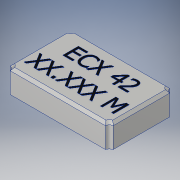
# Autodesk Inventor part: Crystal_ECX-42
Saved by Autodesk Inventor 2017 (Build 210142000, 142)
## iProperties
Created: 2016-08-15
Part Number: Crystal_ECX-42
Material: Aluminum 6061
Document SubType Name: Modeling
Designer: Bradley
Density: 2.7 g/cm^3
Appearance: Aluminum - Flat
Author: Bradley
Autodesk Inventor part; units mm, degrees
ref_plane "YZ Plane" through (0, 0, 0) normal (1, 0, 0) x (0, 1, 0)
ref_plane "XZ Plane" through (0, 0, 0) normal (0, 1, 0) x (-1, 0, 0)
ref_plane "XY Plane" through (0, 0, 0) normal (0, 0, 1) x (1, 0, 0)
sketch "Sketch1" plane through (0, 0, 0) normal (0, 1, 0) x (-1, 0, 0)
  line L0 (-2, 1.25) -> (2, 1.25)
  line L1 (2, 1.25) -> (2, -1.25)
  line L2 (2, -1.25) -> (-2, -1.25)
  line L3 (-2, -1.25) -> (-2, 1.25)
  line L4 (-2, 1.25) -> (2, -1.25) construction
  line L5 (2, 1.25) -> (-2, -1.25) construction
  arc A0 (2, -1.1) -> (1.85, -1.25) centre (2, -1.25) ccw
  arc A1 (-1.85, -1.25) -> (-2, -1.1) centre (-2, -1.25) ccw
  arc A2 (-2, 1.1) -> (-1.85, 1.25) centre (-2, 1.25) ccw
  arc A3 (1.85, 1.25) -> (2, 1.1) centre (2, 1.25) ccw
  point P0 (0, 0)
  dimension "d0" = 4
  dimension "d1" = 2.5
  dimension "d4" = 0.15
  constraints: 12 end point, 8 point on circle, 8 point on line, 4 centre point, 4 coincident, 3 equal radius, 2 midpoint, 2 parallel, 1 horizontal, 1 perpendicular
  measures "d0" distance of L1.end L2.end
  measures "d1" distance of L0.end L1.end
  measures "d4" radius of A0
extrude "Extrusion1" add sketch "Sketch1" along normal mid plane 0.9 contours L0 A3 L1 A0 L2 A1 L3 A2
chamfer "Chamfer1" distance 0.1 angle 45 8 edges at (0, 0.45, 1.25) (-1.8939, 0.45, 1.1439) (-2, 0.45, 0) (-1.8939, 0.45, -1.1439) (0, 0.45, -1.25) (1.8939, 0.45, -1.1439) (2, 0.45, 0) (1.8939, 0.45, 1.1439)
sketch "Sketch2" plane through (0, -0.45, 0) normal (0, -1, 0) x (1, 0, 0)
  line L0 (-2, 1.1) -> (-2, -1.1) projected
  arc A0 (-1.85, -1.25) -> (-2, -1.1) centre (-2, -1.25) ccw projected
  line L1 (-1.85, -1.25) -> (1.85, -1.25) projected
  arc A1 (2, -1.1) -> (1.85, -1.25) centre (2, -1.25) ccw projected
  line L2 (2, -1.1) -> (2, 1.1) projected
  arc A2 (1.85, 1.25) -> (2, 1.1) centre (2, 1.25) ccw projected
  line L3 (1.85, 1.25) -> (-1.85, 1.25) projected
  arc A3 (-2, 1.1) -> (-1.85, 1.25) centre (-2, 1.25) ccw projected
  arc A4 (-1.85, -1.25) -> (-2, -1.1) centre (-2, -1.25) ccw projected
  line L4 (-1.9612, -1.1051) -> (-1.9, -1.0439)
  line L5 (-1.9, 1.0439) -> (-1.9612, 1.1051)
  arc A5 (-2, 1.1) -> (-1.85, 1.25) centre (-2, 1.25) ccw projected
  line L6 (-1.8551, 1.2112) -> (-1.7939, 1.15)
  line L7 (-1.7939, 1.15) -> (-1, 1.15)
  line L8 (-1, -1.15) -> (-1.7939, -1.15)
  line L9 (-1.7939, -1.15) -> (-1.8551, -1.2112)
  arc A6 (1.85, 1.25) -> (2, 1.1) centre (2, 1.25) ccw projected
  line L10 (1.8551, 1.2112) -> (1.7939, 1.15)
  line L11 (1.7939, 1.15) -> (1, 1.15)
  line L12 (1, -1.15) -> (1.7939, -1.15)
  line L13 (1.7939, -1.15) -> (1.8551, -1.2112)
  arc A7 (2, -1.1) -> (1.85, -1.25) centre (2, -1.25) ccw projected
  line L14 (1.9612, -1.1051) -> (1.9, -1.0439)
  line L15 (1.9, 1.0439) -> (1.9612, 1.1051)
  line L16 (-2, 1.25) -> (-1.8939, 1.1439) construction
  line L17 (1.85, 1.25) -> (-1.85, 1.25) construction
  line L18 (-2, -1.25) -> (-1.8939, -1.1439) construction
  line L19 (-1.9, 1.0439) -> (-1.9, 0.35)
  line L20 (-1.9, 0.35) -> (-1, 0.35)
  line L21 (-1, 0.35) -> (-1, 1.15)
  line L22 (-1.9, -1.0439) -> (-1.9, -0.35)
  line L23 (-1.9, -0.35) -> (-1, -0.35)
  line L24 (-1, -0.35) -> (-1, -1.15)
  line L25 (1.9, -1.0439) -> (1.9, -0.35)
  line L26 (1.9, -0.35) -> (1, -0.35)
  line L27 (1, -0.35) -> (1, -1.15)
  line L28 (1.9, 1.0439) -> (1.9, 0.35)
  line L29 (1.9, 0.35) -> (1, 0.35)
  line L30 (1, 1.15) -> (1, 0.35)
  point P0 (0, 0)
  dimension "d9" = 0.15
  dimension "d15" = 2
  dimension "d16" = 0.7
  dimension "d17" = 0.8
  constraints: 52 end point, 15 equal length, 15 point on circle, 9 point on line, 8 parallel, 8 perpendicular, 1 collinear, 1 vertical, 1 other
  measures "d9" distance between parallel lines of L5 L6
  measures "d15" distance between parallel lines of L30 L21
  measures "d16" distance between parallel lines of L26 L29
  measures "d17" distance of L11.end L29.end
sketch "Sketch3" plane through (0, 0.45, 0) normal (0, 1, 0) x (1, 0, 0)
  line L0 (-1.7709, 1.15) -> (1.7709, 1.15) projected
  arc A0 (-1.9, 1.0209) -> (-1.7709, 1.15) centre (-2, 1.25) ccw projected
  line L1 (-1.9, -1.0209) -> (-1.9, 1.0209) projected
  arc A1 (-1.7709, -1.15) -> (-1.9, -1.0209) centre (-2, -1.25) ccw projected
  line L2 (1.7709, -1.15) -> (-1.7709, -1.15) projected
  arc A2 (1.9, -1.0209) -> (1.7709, -1.15) centre (2, -1.25) ccw projected
  line L3 (1.9, 1.0209) -> (1.9, -1.0209) projected
  arc A3 (1.7709, 1.15) -> (1.9, 1.0209) centre (2, 1.25) ccw projected
  line L4 (1.9, 1.0209) -> (1.9, -1.0209) construction
  line L5 (1.9, 0.1868) -> (-1.9, 0.1868) construction
  line L6 (-1.237, 0.1868) -> (-1.237, 0.7868)
  line L7 (-1.237, 0.7868) -> (-0.8616, 0.7868)
  line L8 (-0.8616, 0.7868) -> (-0.8616, 0.7158)
  line L9 (-0.8616, 0.7158) -> (-1.1572, 0.7158)
  line L10 (-1.1572, 0.7158) -> (-1.1572, 0.5514)
  line L11 (-1.1572, 0.5514) -> (-0.8815, 0.5514)
  line L12 (-0.8815, 0.5514) -> (-0.8815, 0.4804)
  line L13 (-0.8815, 0.4804) -> (-1.1572, 0.4804)
  line L14 (-1.1572, 0.4804) -> (-1.1572, 0.2577)
  line L15 (-1.1572, 0.2577) -> (-0.8616, 0.2577)
  line L16 (-0.8616, 0.2577) -> (-0.8616, 0.1868)
  line L17 (-0.8616, 0.1868) -> (-1.237, 0.1868)
  spline S0 degree 2 poles (-0.5397, 0.1761) (-0.5981, 0.1761) (-0.6968, 0.2154) (-0.7327, 0.2548) knots 0 0 0 1 2 2 2
  spline S1 degree 2 poles (-0.7327, 0.2548) (-0.7687, 0.2937) (-0.8081, 0.4104) (-0.8081, 0.4863) knots 0 0 0 1 2 2 2
  spline S2 degree 2 poles (-0.8081, 0.4863) (-0.8081, 0.5616) (-0.7697, 0.6735) (-0.7332, 0.7148) knots 0 0 0 1 2 2 2
  spline S3 degree 2 poles (-0.7332, 0.7148) (-0.6972, 0.7552) (-0.599, 0.7975) (-0.5382, 0.7975) knots 0 0 0 1 2 2 2
  spline S4 degree 2 poles (-0.5382, 0.7975) (-0.5081, 0.7975) (-0.4551, 0.7887) (-0.4327, 0.7819) knots 0 0 0 1 2 2 2
  spline S5 degree 2 poles (-0.4327, 0.7819) (-0.4133, 0.7756) (-0.3729, 0.7576) (-0.353, 0.7469) knots 0 0 0 1 2 2 2
  line L18 (-0.353, 0.7469) -> (-0.353, 0.6506)
  line L19 (-0.353, 0.6506) -> (-0.3593, 0.6506)
  spline S6 degree 2 poles (-0.3593, 0.6506) (-0.37, 0.6603) (-0.4031, 0.6876) (-0.4269, 0.7007) knots 0 0 0 1 2 2 2
  spline S7 degree 2 poles (-0.4269, 0.7007) (-0.4498, 0.7133) (-0.5037, 0.7294) (-0.5387, 0.7294) knots 0 0 0 1 2 2 2
  spline S8 degree 2 poles (-0.5387, 0.7294) (-0.5771, 0.7294) (-0.6457, 0.6978) (-0.6715, 0.6676) knots 0 0 0 1 2 2 2
  spline S9 degree 2 poles (-0.6715, 0.6676) (-0.6968, 0.637) (-0.725, 0.5441) (-0.725, 0.4863) knots 0 0 0 1 2 2 2
  spline S10 degree 2 poles (-0.725, 0.4863) (-0.725, 0.4245) (-0.6953, 0.3355) (-0.6695, 0.3049) knots 0 0 0 1 2 2 2
  spline S11 degree 2 poles (-0.6695, 0.3049) (-0.6442, 0.2752) (-0.5767, 0.2451) (-0.5387, 0.2451) knots 0 0 0 1 2 2 2
  spline S12 degree 2 poles (-0.5387, 0.2451) (-0.5042, 0.2451) (-0.4454, 0.2621) (-0.4225, 0.2748) knots 0 0 0 1 2 2 2
  spline S13 degree 2 poles (-0.4225, 0.2748) (-0.4006, 0.2874) (-0.3681, 0.3137) (-0.3588, 0.3229) knots 0 0 0 1 2 2 2
  line L20 (-0.3588, 0.3229) -> (-0.353, 0.3229)
  line L21 (-0.353, 0.3229) -> (-0.353, 0.2276)
  spline S14 degree 2 poles (-0.353, 0.2276) (-0.3729, 0.2184) (-0.4079, 0.2013) (-0.4327, 0.1936) knots 0 0 0 1 2 2 2
  spline S15 degree 2 poles (-0.4327, 0.1936) (-0.459, 0.1848) (-0.5037, 0.1761) (-0.5397, 0.1761) knots 0 0 0 1 2 2 2
  line L22 (0.1361, 0.1868) -> (0.0447, 0.1868)
  line L23 (0.0447, 0.1868) -> (-0.1011, 0.426)
  line L24 (-0.1011, 0.426) -> (-0.2499, 0.1868)
  line L25 (-0.2499, 0.1868) -> (-0.336, 0.1868)
  line L26 (-0.336, 0.1868) -> (-0.1449, 0.4872)
  line L27 (-0.1449, 0.4872) -> (-0.3301, 0.7868)
  line L28 (-0.3301, 0.7868) -> (-0.2387, 0.7868)
  line L29 (-0.2387, 0.7868) -> (-0.0958, 0.5519)
  line L30 (-0.0958, 0.5519) -> (0.0501, 0.7868)
  line L31 (0.0501, 0.7868) -> (0.1361, 0.7868)
  line L32 (0.1361, 0.7868) -> (-0.0515, 0.4911)
  line L33 (-0.0515, 0.4911) -> (0.1361, 0.1868)
  line L34 (0.8271, 0.3929) -> (0.7556, 0.3929)
  line L35 (0.7556, 0.3929) -> (0.7556, 0.1868)
  line L36 (0.7556, 0.1868) -> (0.6783, 0.1868)
  line L37 (0.6783, 0.1868) -> (0.6783, 0.3929)
  line L38 (0.6783, 0.3929) -> (0.4133, 0.3929)
  line L39 (0.4133, 0.3929) -> (0.4133, 0.4775)
  line L40 (0.4133, 0.4775) -> (0.6817, 0.7868)
  line L41 (0.6817, 0.7868) -> (0.7556, 0.7868)
  line L42 (0.7556, 0.7868) -> (0.7556, 0.4576)
  line L43 (0.7556, 0.4576) -> (0.8271, 0.4576)
  line L44 (0.8271, 0.4576) -> (0.8271, 0.3929)
  line L45 (0.6783, 0.4576) -> (0.6783, 0.6919)
  line L46 (0.6783, 0.6919) -> (0.4765, 0.4576)
  line L47 (0.4765, 0.4576) -> (0.6783, 0.4576)
  line L48 (1.2613, 0.1868) -> (0.8912, 0.1868)
  line L49 (0.8912, 0.1868) -> (0.8912, 0.2718)
  spline S16 degree 2 poles (0.8912, 0.2718) (0.9311, 0.3093) (1.0021, 0.3788) (1.0361, 0.4163) knots 0 0 0 1 2 2 2
  spline S17 degree 2 poles (1.0361, 0.4163) (1.1047, 0.4916) (1.1548, 0.5821) (1.1548, 0.6302) knots 0 0 0 1 2 2 2
  spline S18 degree 2 poles (1.1548, 0.6302) (1.1548, 0.6555) (1.1392, 0.6934) (1.1251, 0.7056) knots 0 0 0 1 2 2 2
  spline S19 degree 2 poles (1.1251, 0.7056) (1.111, 0.7177) (1.0741, 0.7299) (1.0517, 0.7299) knots 0 0 0 1 2 2 2
  spline S20 degree 2 poles (1.0517, 0.7299) (1.0303, 0.7299) (0.9865, 0.7192) (0.9666, 0.7109) knots 0 0 0 1 2 2 2
  spline S21 degree 2 poles (0.9666, 0.7109) (0.9496, 0.7041) (0.918, 0.6846) (0.9083, 0.6778) knots 0 0 0 1 2 2 2
  line L50 (0.9083, 0.6778) -> (0.9039, 0.6778)
  line L51 (0.9039, 0.6778) -> (0.9039, 0.7634)
  spline S22 degree 2 poles (0.9039, 0.7634) (0.9287, 0.7756) (1.0177, 0.7994) (1.0575, 0.7994) knots 0 0 0 1 2 2 2
  spline S23 degree 2 poles (1.0575, 0.7994) (1.1417, 0.7994) (1.2365, 0.7104) (1.2365, 0.6346) knots 0 0 0 1 2 2 2
  spline S24 degree 2 poles (1.2365, 0.6346) (1.2365, 0.5991) (1.2199, 0.5398) (1.2053, 0.5145) knots 0 0 0 1 2 2 2
  spline S25 degree 2 poles (1.2053, 0.5145) (1.1908, 0.4882) (1.1485, 0.4367) (1.1251, 0.4119) knots 0 0 0 1 2 2 2
  spline S26 degree 2 poles (1.1251, 0.4119) (1.0872, 0.3705) (0.9943, 0.2821) (0.9666, 0.2563) knots 0 0 0 1 2 2 2
  line L52 (0.9666, 0.2563) -> (1.2613, 0.2563)
  line L53 (1.2613, 0.2563) -> (1.2613, 0.1868)
  line L54 (-1.2936, -0.7914) -> (-1.385, -0.7914)
  line L55 (-1.385, -0.7914) -> (-1.5309, -0.5522)
  line L56 (-1.5309, -0.5522) -> (-1.6797, -0.7914)
  line L57 (-1.6797, -0.7914) -> (-1.7657, -0.7914)
  line L58 (-1.7657, -0.7914) -> (-1.5746, -0.4909)
  line L59 (-1.5746, -0.4909) -> (-1.7599, -0.1914)
  line L60 (-1.7599, -0.1914) -> (-1.6685, -0.1914)
  line L61 (-1.6685, -0.1914) -> (-1.5255, -0.4263)
  line L62 (-1.5255, -0.4263) -> (-1.3797, -0.1914)
  line L63 (-1.3797, -0.1914) -> (-1.2936, -0.1914)
  line L64 (-1.2936, -0.1914) -> (-1.4813, -0.487)
  line L65 (-1.4813, -0.487) -> (-1.2936, -0.7914)
  line L66 (-0.8147, -0.7914) -> (-0.9061, -0.7914)
  line L67 (-0.9061, -0.7914) -> (-1.0519, -0.5522)
  line L68 (-1.0519, -0.5522) -> (-1.2007, -0.7914)
  line L69 (-1.2007, -0.7914) -> (-1.2868, -0.7914)
  line L70 (-1.2868, -0.7914) -> (-1.0957, -0.4909)
  line L71 (-1.0957, -0.4909) -> (-1.281, -0.1914)
  line L72 (-1.281, -0.1914) -> (-1.1895, -0.1914)
  line L73 (-1.1895, -0.1914) -> (-1.0466, -0.4263)
  line L74 (-1.0466, -0.4263) -> (-0.9007, -0.1914)
  line L75 (-0.9007, -0.1914) -> (-0.8147, -0.1914)
  line L76 (-0.8147, -0.1914) -> (-1.0024, -0.487)
  line L77 (-1.0024, -0.487) -> (-0.8147, -0.7914)
  line L78 (-0.6387, -0.7914) -> (-0.7349, -0.7914)
  line L79 (-0.7349, -0.7914) -> (-0.7349, -0.6767)
  line L80 (-0.7349, -0.6767) -> (-0.6387, -0.6767)
  line L81 (-0.6387, -0.6767) -> (-0.6387, -0.7914)
  line L82 (-0.0858, -0.7914) -> (-0.1772, -0.7914)
  line L83 (-0.1772, -0.7914) -> (-0.3231, -0.5522)
  line L84 (-0.3231, -0.5522) -> (-0.4719, -0.7914)
  line L85 (-0.4719, -0.7914) -> (-0.5579, -0.7914)
  line L86 (-0.5579, -0.7914) -> (-0.3669, -0.4909)
  line L87 (-0.3669, -0.4909) -> (-0.5521, -0.1914)
  line L88 (-0.5521, -0.1914) -> (-0.4607, -0.1914)
  line L89 (-0.4607, -0.1914) -> (-0.3177, -0.4263)
  line L90 (-0.3177, -0.4263) -> (-0.1719, -0.1914)
  line L91 (-0.1719, -0.1914) -> (-0.0858, -0.1914)
  line L92 (-0.0858, -0.1914) -> (-0.2735, -0.487)
  line L93 (-0.2735, -0.487) -> (-0.0858, -0.7914)
  line L94 (0.3931, -0.7914) -> (0.3017, -0.7914)
  line L95 (0.3017, -0.7914) -> (0.1558, -0.5522)
  line L96 (0.1558, -0.5522) -> (0.0071, -0.7914)
  line L97 (0.0071, -0.7914) -> (-0.079, -0.7914)
  line L98 (-0.079, -0.7914) -> (0.1121, -0.4909)
  line L99 (0.1121, -0.4909) -> (-0.0732, -0.1914)
  line L100 (-0.0732, -0.1914) -> (0.0182, -0.1914)
  line L101 (0.0182, -0.1914) -> (0.1612, -0.4263)
  line L102 (0.1612, -0.4263) -> (0.3071, -0.1914)
  line L103 (0.3071, -0.1914) -> (0.3931, -0.1914)
  line L104 (0.3931, -0.1914) -> (0.2054, -0.487)
  line L105 (0.2054, -0.487) -> (0.3931, -0.7914)
  line L106 (0.872, -0.7914) -> (0.7806, -0.7914)
  line L107 (0.7806, -0.7914) -> (0.6348, -0.5522)
  line L108 (0.6348, -0.5522) -> (0.486, -0.7914)
  line L109 (0.486, -0.7914) -> (0.3999, -0.7914)
  line L110 (0.3999, -0.7914) -> (0.591, -0.4909)
  line L111 (0.591, -0.4909) -> (0.4058, -0.1914)
  line L112 (0.4058, -0.1914) -> (0.4972, -0.1914)
  line L113 (0.4972, -0.1914) -> (0.6401, -0.4263)
  line L114 (0.6401, -0.4263) -> (0.786, -0.1914)
  line L115 (0.786, -0.1914) -> (0.872, -0.1914)
  line L116 (0.872, -0.1914) -> (0.6844, -0.487)
  line L117 (0.6844, -0.487) -> (0.872, -0.7914)
  line L118 (1.7083, -0.7914) -> (1.6286, -0.7914)
  line L119 (1.6286, -0.7914) -> (1.6286, -0.2746)
  line L120 (1.6286, -0.2746) -> (1.472, -0.6261)
  line L121 (1.472, -0.6261) -> (1.4234, -0.6261)
  line L122 (1.4234, -0.6261) -> (1.2683, -0.2746)
  line L123 (1.2683, -0.2746) -> (1.2683, -0.7914)
  line L124 (1.2683, -0.7914) -> (1.1939, -0.7914)
  line L125 (1.1939, -0.7914) -> (1.1939, -0.1914)
  line L126 (1.1939, -0.1914) -> (1.3028, -0.1914)
  line L127 (1.3028, -0.1914) -> (1.4526, -0.5255)
  line L128 (1.4526, -0.5255) -> (1.5975, -0.1914)
  line L129 (1.5975, -0.1914) -> (1.7083, -0.1914)
  line L130 (1.7083, -0.1914) -> (1.7083, -0.7914)
  point P0 (0, 0)
  constraints: 2 end point, 2 point on line, 1 horizontal, 1 perpendicular
extrude "Extrusion3" add sketch "Sketch3" along normal blind 0.01 contours L6 L7 L8 L9 L10 L11 L12 L13 L14 L15 L16 L17 | S0 S1 S2 S3 S4 S5 L18 L19 S6 S7 S8 S9 S10 S11 S12 S13 L20 L21 S14 S15 | L22 L23 L24 L25 L26 L27 L28 L29 L30 L31 L32 L33 | L34 L35 L36 L37 L38 L39 L40 L41 L42 L43 L44 | L48 L49 S16 S17 S18 S19 S20 S21 L50 L51 S22 S23 S24 S25 S26 L52 L53 | L54 L55 L56 L57 L58 L59 L60 L61 L62 L63 L64 L65 | L66 L67 L68 L69 L70 L71 L72 L73 L74 L75 L76 L77 | L78 L79 L80 L81 | L82 L83 L84 L85 L86 L87 L88 L89 L90 L91 L92 L93 | L94 L95 L96 L97 L98 L99 L100 L101 L102 L103 L104 L105 | L106 L107 L108 L109 L110 L111 L112 L113 L114 L115 L116 L117 | L118 L119 L120 L121 L122 L123 L124 L125 L126 L127 L128 L129 L130
extrude "Extrusion4" add sketch "Sketch2" along normal blind 0.01 contours A3 L6 L7 L21 L20 L19 L5 | L4 L22 L23 L24 L8 L9 A0 | A2 L15 L28 L29 L30 L11 L10 | L13 L12 L27 L26 L25 L14 A1
body "Solid1"
